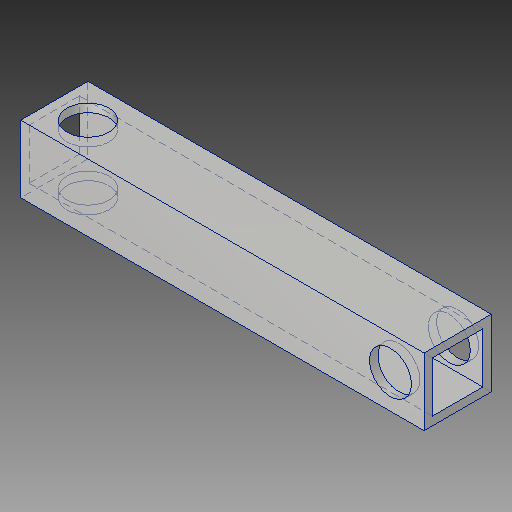
# Autodesk Inventor part: Coupler
Saved by Autodesk Inventor 2019 (Build 230136000, 136)
## iProperties
Created: 2018-09-28
Part Number: Coupler
Material: Aluminum 6061
Document SubType Name: Modeling
Designer: Adhik
Density: 2.7 g/cm^3
Appearance: Aluminum - Flat
Mass: 109.356 g
Surface Area: 267.112 cm^2
Volume: 40.5023 cm^3
Author: Adhik
Autodesk Inventor part; units mm, degrees
ref_plane "YZ Plane" through (0, 0, 0) normal (1, 0, 0) x (0, 1, 0)
ref_plane "XZ Plane" through (0, 0, 0) normal (0, 1, 0) x (-1, 0, 0)
ref_plane "XY Plane" through (0, 0, 0) normal (0, 0, 1) x (1, 0, 0)
sketch "Sketch1" plane through (0, 0, 0) normal (1, 0, 0) x (0, 1, 0)
  line L0 (-17.78, 0) -> (17.78, 0) construction
  line L1 (0, -17.78) -> (0, 17.78) construction
  line L2 (9.525, 9.525) -> (-9.525, 9.525)
  line L3 (-9.525, 9.525) -> (-9.525, -9.525)
  line L4 (-9.525, -9.525) -> (9.525, -9.525)
  line L5 (9.525, -9.525) -> (9.525, 9.525)
  line L6 (12.7, 12.7) -> (-12.7, 12.7)
  line L7 (-12.7, 12.7) -> (-12.7, -12.7)
  line L8 (-12.7, -12.7) -> (12.7, -12.7)
  line L9 (12.7, -12.7) -> (12.7, 12.7)
  point P0 (0, 0)
  point P1 (0, 12.7)
  point P2 (0, 9.525)
  point P3 (12.7, 0)
  point P4 (9.525, 0)
  dimension "d0" = 3.175
  dimension "d1" = 25.4
  constraints: 16 end point, 4 midpoint, 4 parallel, 4 perpendicular, 4 point on line, 2 horizontal
  measures "d0" distance between parallel lines of L6 L2
  measures "d1" distance of L6.start L6.end
extrude "Extrusion1" add sketch "Sketch1" along normal mid plane 152.4
sketch "Sketch2" plane through (-76.2, -12.7, 12.7) normal (0, 0, 1) x (1, 0, 0)
  line L0 (76.2, -5.08) -> (76.2, 30.48) construction
  line L1 (-30.48, 12.7) -> (182.88, 12.7) construction
  circle A0 centre (139.7, 12.7) radius 7.9375
  line L2 (152.4, 25.4) -> (152.4, 0) construction
  point P0 (76.2, 12.7)
  dimension "d4" = 15.875
  dimension "d5" = 12.7
  constraints: 1 centre point, 1 point on line
  measures "d4" diameter of A0
  measures "d5" distance from line of L2 A0.centre
extrude "Extrusion2" cut sketch "Sketch2" against normal through all
sketch "Sketch3" plane through (-76.2, 12.7, 12.7) normal (0, 1, 0) x (1, 0, 0)
  line L0 (76.2, 30.48) -> (76.2, -5.08) construction
  line L1 (-30.48, 12.7) -> (182.88, 12.7) construction
  circle A0 centre (12.7, 12.7) radius 7.9375
  line L2 (0, 0) -> (0, 25.4) construction
  point P0 (76.2, 12.7)
  dimension "d8" = 12.7
  dimension "d9" = 15.875
  constraints: 1 centre point, 1 point on line
  measures "d8" distance from line of L2 A0.centre
  measures "d9" diameter of A0
extrude "Extrusion3" cut sketch "Sketch3" against normal through all
body "Solid1"
